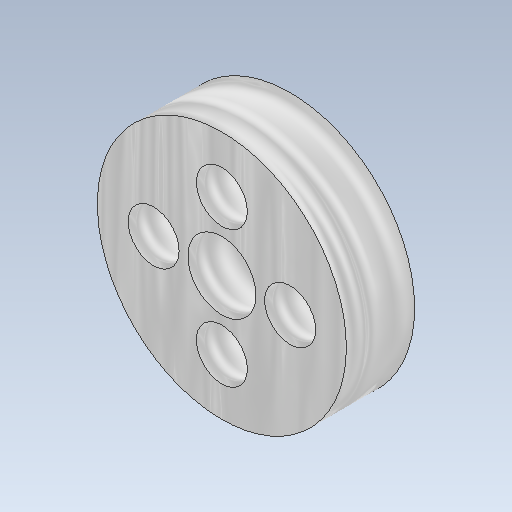
# Autodesk Inventor part: 脚中間フレームカム
Saved by Autodesk Inventor 2020.2 (Build 242310000, 310)
## iProperties
Created: 2020-03-13
Part Number: 脚中間フレームカム
Material: アルミニウム 7075
Document SubType Name: Modeling
Designer: aoyam
Density: 2.81 g/cm^3
Appearance: サテン - ブラシ仕上げ 重厚
Mass: 1.42294 g
Surface Area: 6.3697 cm^2
Volume: 0.506386 cm^3
Author: aoyam
Autodesk Inventor part; units mm, degrees
ref_plane "YZ Plane" through (0, 0, 0) normal (1, 0, 0) x (0, 1, 0)
ref_plane "XZ Plane" through (0, 0, 0) normal (0, 1, 0) x (-1, 0, 0)
ref_plane "XY Plane" through (0, 0, 0) normal (0, 0, 1) x (1, 0, 0)
sketch "スケッチ1" plane through (0, 0, 0) normal (0, 0, 1) x (1, 0, 0)
  line L0 (0, 0) -> (-4, 0) construction
  circle A0 centre (-4, 0) radius 1.495
  line L1 (0, 0) -> (0, -4) construction
  circle A1 centre (0, -4) radius 1.495
  line L2 (0, 0) -> (4, 0) construction
  circle A2 centre (4, 0) radius 1.495
  line L3 (0, 0) -> (0, 4) construction
  circle A3 centre (0, 4) radius 1.495
  line L4 (0, 0) -> (-8.8388, 8.8388) construction
  circle A4 centre (-8.8388, 8.8388) radius 1.5
  line L5 (0, 0) -> (-8.8388, -8.8388) construction
  circle A5 centre (-8.8388, -8.8388) radius 1.5
  line L6 (0, 0) -> (8.8388, -8.8388) construction
  circle A6 centre (8.8388, -8.8388) radius 1.5
  line L7 (0, 0) -> (8.8388, 8.8388) construction
  circle A7 centre (8.8388, 8.8388) radius 1.5
  circle A8 centre (0, 0) radius 7.295
  circle A9 centre (0, 0) radius 15.5
  circle A10 centre (0, 0) radius 1.995
  dimension "d0" = 4
  dimension "d1" = 2.99
  dimension "d4" = 360
  dimension "d6" = 12.5
  dimension "d7" = 3
  dimension "d8" = 45
  dimension "d11" = 360
  dimension "d13" = 1.8
  dimension "d14" = 14.59
  dimension "d15" = 1.5
  dimension "d16" = 3.99
  constraints: 16 end point, 13 coincident, 11 centre point, 1 horizontal, 40 other
  measures "d0" distance of L0.start L0.end
  measures "d1" diameter of A0
  measures "d6" distance of L3.start L4.end
  measures "d7" diameter of A4
  measures "d8" angle of L4 L0
  measures "d14" diameter of A8
  measures "d16" diameter of A10
extrude "押し出し1" add sketch "スケッチ1" along normal blind 4 contours A8
